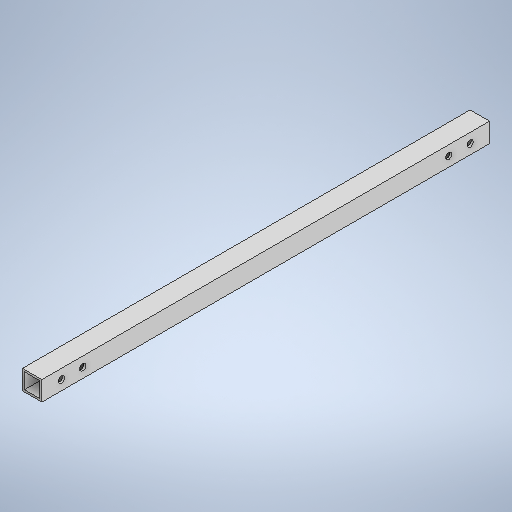
# Autodesk Inventor part: kaku_1010_230
Saved by Autodesk Inventor 2025.1 (Build 291241000, 241)
## iProperties
Created: 2024-11-05
Part Number: kaku_1010_230
Material: 一般
Document SubType Name: Modeling
Designer: yuki0520
Density: 1 g/cm^3
Appearance: 既定
Author: yuki0520
Autodesk Inventor part; units mm, degrees
ref_plane "YZ Plane" through (0, 0, 0) normal (1, 0, 0) x (0, 1, 0)
ref_plane "XZ Plane" through (0, 0, 0) normal (0, 1, 0) x (-1, 0, 0)
ref_plane "XY Plane" through (0, 0, 0) normal (0, 0, 1) x (1, 0, 0)
sketch "スケッチ1" plane through (0, 0, 0) normal (0, 0, 1) x (1, 0, 0)
  line L0 (5, -5) -> (-5, -5)
  line L1 (-5, -5) -> (-5, 5)
  line L2 (-5, 5) -> (5, 5)
  line L3 (5, 5) -> (5, -5)
  line L4 (5, -5) -> (-5, 5) construction
  line L5 (-5, -5) -> (5, 5) construction
  line L6 (4, 4) -> (-4, 4)
  line L7 (-4, 4) -> (-4, -4)
  line L8 (-4, -4) -> (4, -4)
  line L9 (4, -4) -> (4, 4)
  point P0 (0, 0)
  dimension "d0" = 10
  dimension "d1" = 10
  dimension "d2" = 1
  constraints: 20 end point, 4 parallel, 2 midpoint, 2 perpendicular, 1 horizontal, 3 other
  measures "d0" distance of L1.end L2.end
  measures "d1" distance of L0.end L1.end
  measures "d2" distance between parallel lines of L2 L6
extrude "押し出し1" add sketch "スケッチ1" along normal blind 230
sketch "スケッチ2" plane through (5, -5, 0) normal (1, 0, 0) x (0, 0, -1)
  line L0 (0, 0) -> (0, 10) projected
  line L1 (0, 10) -> (-230, 10) projected
  line L2 (-230, 0) -> (-230, 10) projected
  line L3 (0, 0) -> (-230, 0) projected
  line L4 (-230, 5) -> (0, 5)
  point P0 (-220, 5)
  point P1 (-10, 5)
  point P2 (-209, 5)
  point P3 (-21, 5)
  point P4 (-115, 5)
  dimension "d5" = 210
  dimension "d6" = 10
  dimension "d14" = 188
  dimension "d15" = 94
  constraints: 4 point on line, 2 end point, 2 midpoint, 1 horizontal
  measures "d5" distance of point (-10, 5) point (-220, 5)
  measures "d6" distance from line of L0 point (-10, 5)
  measures "d14" distance of point (-21, 5) point (-209, 5)
  measures "d15" distance of point (-115, 5) point (-209, 5)
hole "穴1" at (5, 0, 220) at (5, 0, 10) at (5, 0, 209) at (5, 0, 21) direction (-1, 0, 0) diameter 3.3 end through all
equation "\"d15\" = 0.5 * d14"
